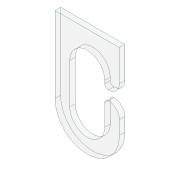
# Autodesk Inventor part: uhook
Saved by Autodesk Inventor 2020 (Build 240168000, 168)
## iProperties
Created: 2021-06-22
Part Number: uhook
Material: Generic
Document SubType Name: Modeling
Designer: Aidan Lee
Density: 1 g/cm^3
Appearance: Clear
Author: Aidan Lee
Autodesk Inventor part; units mm, degrees
ref_plane "YZ Plane" through (0, 0, 0) normal (1, 0, 0) x (0, 1, 0)
ref_plane "XZ Plane" through (0, 0, 0) normal (0, 1, 0) x (-1, 0, 0)
ref_plane "XY Plane" through (0, 0, 0) normal (0, 0, 1) x (1, 0, 0)
sketch "Sketch1" plane through (0, 0, 0) normal (0, 0, 1) x (1, 0, 0)
  line L0 (-1.5, 4) -> (1.5, 4) construction
  line L1 (1.5, 4) -> (1.5, -4) construction
  line L2 (1.5, -4) -> (-1.5, -4) construction
  line L3 (-1.5, -4) -> (-1.5, 4) construction
  line L4 (9.5, 2.5) -> (9.5, -29) construction
  line L5 (9.5, -29) -> (-9.5, -29) construction
  line L6 (-9.5, -29) -> (-9.5, 2.5)
  arc A0 (-9.5, -19.5) -> (9.5, -19.5) centre (0, -19.5) ccw
  arc A1 (-17.5, -19.5) -> (17.5, -19.5) centre (0, -19.5) ccw
  line L7 (11.5, -1) -> (20.6171, -1) construction
  line L8 (17.5, 5) -> (17.5, 22)
  line L9 (-17.5, -19.5) -> (-17.5, 22)
  line L10 (9.5, 1) -> (9.5, 2.5)
  line L11 (0, -37) -> (17.5, -37) construction
  arc A2 (11.5, -1) -> (17.5, 5) centre (11.5, 5) ccw
  arc A3 (9.5, 1) -> (11.5, -1) centre (11.5, 1) ccw
  line L12 (11.4283, -3.5) -> (20.9038, -3.5) construction
  arc A4 (17.5, -12) -> (11.5, -6) centre (11.5, -12) ccw
  arc A5 (11.5, -6) -> (9.5, -8) centre (11.5, -8) ccw
  line L13 (9.5, -8) -> (9.5, -19.5)
  line L14 (17.5, -19.5) -> (17.5, -12)
  line L15 (-17.5, 22) -> (17.5, 22)
  line L16 (-22.1996, 12) -> (26.487, 12) construction
  arc A6 (9.5, 2.5) -> (-9.5, 2.5) centre (0, 2.5) ccw
  point P0 (0, 0)
  point P1 (0, -4)
  point P2 (-1.5, 0)
  point P3 (0, -29)
  point P4 (0, 12)
  dimension "d0" = 8
  dimension "d1" = 3
  dimension "extra" = 25
  dimension "d4" = 8
  dimension "d6" = 8
  dimension "d10" = 4
  dimension "d11" = 2.5
  dimension "d12" = 3.5
  dimension "d18" = 8
  dimension "d21" = 10
  dimension "d22" = 35
  constraints: 35 end point, 17 point on circle, 7 centre point, 7 vertical alignment, 5 horizontal, 5 horizontal alignment, 5 symmetric about line, 5 tangent, 4 parallel, 3 midpoint, 3 point on line, 2 collinear, 2 perpendicular, 1 coincident, 1 vertical, 2 other
  measures "d0" distance of L2.end L0.start
  measures "d1" distance of L1.end L2.end
  measures "extra" distance between parallel lines of L5 L2
  measures "d4" distance between parallel lines of L6 L3
  measures "d6" radial gap between concentric circles of A1 A0
  measures "d10" distance of A2.centre A3.centre
  measures "d11" distance between parallel lines of L12 L7
  measures "d12" distance from line of point (0, 0) L12
  measures "d18" distance from line of L16.start L0
  measures "d21" vertical distance of L9.end point (0, 12)
  measures "d22" distance between parallel lines of L8 L9
extrude "Extrusion1" add sketch "Sketch1" along normal blind 3
body "Solid1"
